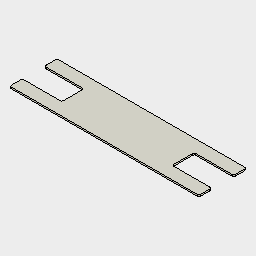
Slide Holder (Autodesk Fusion 360 design; units mm, degrees)
Autodesk Fusion 360 part; units mm, degrees
sketch "Sketch1" plane through (0, 0, 0) normal (0, 0, 1) x (1, 0, 0)
  line L0 (-60, 15) -> (60, 15)
  line L1 (60, 15) -> (60, 7)
  line L2 (60, 7) -> (-60, 7)
  line L3 (-60, 7) -> (-60, 15)
  line L4 (-60, -7) -> (60, -7)
  line L5 (60, -7) -> (60, -15)
  line L6 (60, -15) -> (-60, -15)
  line L7 (-60, -15) -> (-60, -7)
  line L8 (-35, 7) -> (35, 7)
  line L9 (35, 7) -> (35, -7)
  line L10 (35, -7) -> (-35, -7)
  line L11 (-35, -7) -> (-35, 7)
  line L12 (-25, 8) -> (25, 8)
  line L13 (25, 8) -> (25, -8)
  line L14 (25, -8) -> (-25, -8)
  line L15 (-25, -8) -> (-25, 8)
  dimension "d24" = 120
  dimension "d25" = 8
  dimension "d26" = 8
  dimension "d27" = 30
  dimension "d28" = 70
  dimension "d29" = 25
  dimension "d30" = 50
  dimension "d32" = 7
  dimension "d33" = 10
  dimension "d34" = 60
  dimension "d35" = 15
  dimension "d37" = 1
  measures "d24" distance of L0.start L0.end
  measures "d25" distance of L0.start L2.end
  measures "d26" distance of L4.start L6.end
  measures "d27" distance of L0 L6
  measures "d28" distance of L8.start L8.end
  measures "d29" distance of L1 L9
  measures "d30" distance of L12.start L12.end
  measures "d32" distance of L0 L12
  measures "d33" distance of L11 L15
  measures "d34" distance of origin L3
  measures "d35" distance of origin L0
  measures "d37" distance of L10 L14
extrude "Extrude1" add sketch "Sketch1" along normal blind 1
fillet "Fillet1" radius 1 12 edges at (-60, 15, 0.5) (-60, 7, 0.5) (-60, -7, 0.5) (-60, -15, 0.5) (-35, 7, 0.5) (-35, -7, 0.5) (60, -15, 0.5) (60, -7, 0.5) (35, 7, 0.5) (35, -7, 0.5) (60, 7, 0.5) (60, 15, 0.5)
equation "d26 = d25"
equation "d34 = d24 / 2"
equation "d35 = d27 / 2"
